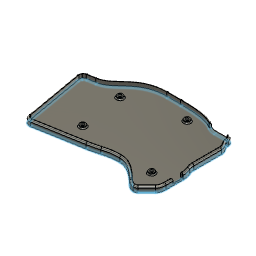
case (Autodesk Fusion 360 design; units mm, degrees)
Autodesk Fusion 360 part; units mm, degrees
note: some values were not read from the file. Set by a fixed rule: the direction of a hole.
sketch "holes" plane through (0, 0, 0) normal (0, 1, 0) x (1, 0, 0)
  circle A0 centre (50.040422, 45.440379) radius 3
  circle A1 centre (43.351531, 91.955525) radius 3
  circle A2 centre (130.099984, 39.118187) radius 3
  circle A3 centre (100.999988, 106.018187) radius 3
  line L0 (119.54041, 105.410769) -> (119.54041, 115.410769)
  line L1 (153.850239, 50.591394) -> (146.676652, 50.591394)
  line L2 (119.54041, 115.410769) -> (139.54041, 115.410769)
  line L3 (146.676652, 50.591394) -> (146.676652, 40.591394)
  line L4 (139.54041, 105.410769) -> (119.54041, 105.410769)
  line L5 (153.850239, 40.591394) -> (153.850239, 50.591394)
  line L6 (146.676652, 40.591394) -> (153.850239, 40.591394)
  line L7 (139.54041, 115.410769) -> (139.54041, 105.410769)
extrude "Extrude7" add sketch "holes" along normal blind 4 contours A0 | A1 | A2 | A3 picked at (49.284643, 47.135619) picked at (42.565449, 90.461331) picked at (132.445357, 39.165571) picked at (101.826227, 105.454867) makes body 1 at (51.274283, 2.666667, -48.174896) makes body 2 at (133.096255, 2.666667, -38.96865) makes body 3 at (46.347802, 2.666667, -91.805987) makes body 4 at (103.996259, 2.666667, -105.86865)
hole "Hole1" at (100.999988, 0, -106.018187) at (43.351531, 0, -91.955525) at (50.040422, 0, -45.440379) at (130.099984, 0, -39.118187) direction (0, 1, 0) diameter 3.3 depth 15 tip angle 180 bodies 1 4 2 3
sketch "outline" plane through (0, 0, 0) normal (0, 1, 0) x (1, 0, 0)
  spline S0 degree 3 poles (147.603738, 59.518008) (146.881991, 61.213684) (146.199862, 62.815653) (146.199862, 66.008223) knots 0 0 0 0 1 1 1 1
  line L0 (146.199862, 66.008223) -> (146.199862, 95.722689)
  spline S1 degree 3 poles (146.199862, 95.722689) (146.199862, 97.999035) (144.934803, 99.77514) (143.818612, 101.342328) (142.857757, 102.691416) (141.949992, 103.965769) (141.949992, 105.358104) knots 2 2 2 2 3 3 3 4 4 4 4
  line L1 (141.949992, 105.358104) -> (141.949992, 107.018123)
  spline S2 degree 3 poles (141.949992, 107.018123) (141.949992, 108.782701) (140.514421, 110.2181) (138.749843, 110.2181) knots 5 5 5 5 6 6 6 6
  line L2 (138.749843, 110.2181) -> (125.549959, 110.2181)
  spline S3 degree 3 poles (125.549959, 110.2181) (121.616005, 110.2181) (119.951335, 111.131223) (117.647255, 112.394711) knots 7 7 7 7 8 8 8 8
  spline S4 degree 3 poles (117.647255, 112.394711) (113.165875, 114.852443) (107.028437, 118.218129) (81.750049, 118.218129) knots 8 8 8 8 9 9 9 9
  line L3 (81.750049, 118.218129) -> (66.990398, 118.217956)
  spline S5 degree 3 poles (66.990398, 118.217956) (48.948261, 117.923228) (40.458988, 110.069833) (32.969219, 103.14084) (27.75056, 98.312914) (23.243542, 94.143457) (16.261884, 93.030863) knots 10 10 10 10 11 11 11 12 12 12 12
  line L4 (16.261884, 93.030863) -> (7.644839, 91.511404)
  ellipse E0 centre (8.763061, 86.940358) end of major axis (11.313219, 82.922603) minor radius 4.306681 (7.644839, 91.511404) -> (5.095124, 89.887041) ccw
  ellipse E1 centre (9.103428, 87.448817) end of major axis (13.733249, 86.415108) minor radius 4.300094 (5.095124, 89.887041) -> (4.440728, 86.935456) ccw
  line L5 (4.440728, 86.935456) -> (15.467273, 24.400083)
  spline S6 degree 3 poles (15.467273, 24.400083) (15.80093, 22.508381) (17.435628, 21.13551) (19.354374, 21.13551) (19.583818, 21.13551) (19.8155, 21.155836) (20.043393, 21.196144) knots 16 16 16 16 17 17 17 18 18 18 18
  line L6 (20.043393, 21.196144) -> (70.514731, 30.095514)
  spline S7 degree 3 poles (70.514731, 30.095514) (75.972968, 31.05773) (79.769808, 32.108828) (83.119819, 33.036248) knots 19 19 19 19 20 20 20 20
  spline S8 degree 3 poles (83.119819, 33.036248) (88.53327, 34.53452) (92.808978, 35.718255) (101.339551, 35.718255) knots 20 20 20 20 21 21 21 21
  spline S9 degree 3 poles (101.339551, 35.718255) (111.773711, 35.629027) (121.148505, 26.837832) (127.99391, 20.41893) knots 21 21 21 21 22 22 22 22
  spline S10 degree 3 poles (127.99391, 20.41893) (128.488281, 19.95522) (128.967149, 19.50598) (129.430515, 19.075687) knots 22 22 22 22 23 23 23 23
  spline S11 degree 3 poles (129.430515, 19.075687) (130.520199, 17.98187) (133.15673, 15.944785) (135.470112, 15.94444) knots 23 23 23 23 24 24 24 24
  spline S12 degree 3 poles (135.470112, 15.94444) (135.470456, 15.94444) (135.470456, 15.94444) (135.470801, 15.94444) (136.374794, 15.94444) (137.172678, 16.252776) (137.793829, 16.851534) knots 24 24 24 24 25 25 25 26 26 26 26
  line L7 (137.793829, 16.851534) -> (147.057001, 26.118152)
  spline S13 degree 3 poles (147.057001, 26.118152) (149.010026, 27.990906) (149.268408, 30.899255) (149.275298, 33.227451) knots 27 27 27 27 28 28 28 28
  line L8 (149.275298, 33.227451) -> (149.275298, 51.551225)
  spline S14 degree 3 poles (149.275298, 51.551225) (149.275298, 55.590944) (148.387153, 57.677293) (147.603738, 59.518008) knots 29 29 29 29 30 30 30 30
  spline S15 degree 3 poles (7.297564, 93.481023) (5.763307, 93.210509) (4.350598, 92.310441) (3.456914, 91.034329) knots 2.78448486 2.78448486 2.78448486 2.78448486 3.50173052 3.50173052 3.50173052 3.50173052
  spline S16 degree 3 poles (3.456914, 91.034329) (2.563151, 89.758126) (2.200589, 88.122569) (2.471108, 86.588186) knots 2.7837328 2.7837328 2.7837328 2.7837328 3.50215444 3.50215444 3.50215444 3.50215444
  line L9 (2.471108, 86.588186) -> (13.497675, 24.052686)
  spline S17 degree 3 poles (13.497675, 24.052686) (13.923121, 21.64058) (15.779485, 19.762796) (18.110966, 19.266153) (18.514055, 19.180288) (18.930917, 19.13551) (19.354374, 19.13551) (19.701936, 19.13551) (20.048463, 19.165998) (20.391728, 19.226712) knots 16 16 16 16 16.85259515 16.85259515 16.85259515 17 17 17 18 18 18 18
  line L10 (20.391728, 19.226712) -> (70.861987, 28.125892)
  spline S18 degree 3 poles (70.861987, 28.125892) (76.409207, 29.103795) (80.303318, 30.1813) (83.6533, 31.108711) knots 19.00000221 19.00000221 19.00000221 19.00000221 19.9999871 19.9999871 19.9999871 19.9999871
  spline S19 degree 3 poles (83.6533, 31.108711) (89.064937, 32.606481) (92.991252, 33.717446) (101.330805, 33.718254) knots 20 20 20 20 20.99965063 20.99965063 20.99965063 20.99965063
  spline S20 degree 3 poles (101.330805, 33.718254) (105.475647, 33.680742) (109.565746, 32.090965) (113.464274, 29.700724) (118.330094, 26.717423) (122.82633, 22.522813) (126.625656, 18.960205) knots 21.00029885 21.00029885 21.00029885 21.00029885 21.44497778 21.44497778 21.44497778 21.99998926 21.99998926 21.99998926 21.99998926
  spline S21 degree 3 poles (126.625656, 18.960205) (127.110442, 18.505485) (127.582537, 18.062588) (128.042517, 17.635267) knots 22 22 22 22 22.98076196 22.98076196 22.98076196 22.98076196
  spline S22 degree 3 poles (128.042517, 17.635267) (128.742667, 16.93793) (129.795646, 16.061685) (131.101379, 15.303235) (132.228147, 14.648739) (133.533208, 14.066903) (135.035069, 13.960088) (135.178323, 13.949899) (135.3233, 13.944462) (135.469814, 13.94444) (135.469864, 13.94444) (135.469913, 13.94444) (135.469963, 13.94444) knots 23.00707695 23.00707695 23.00707695 23.00707695 23.51751165 23.51751165 23.51751165 23.95798579 23.95798579 23.95798579 24 24 24 24.00002146 24.00002146 24.00002146 24.00002146
  spline S23 degree 3 poles (135.469963, 13.94444) (135.470012, 13.94444) (135.470062, 13.94444) (135.470112, 13.94444) (135.470456, 13.94444) (135.470456, 13.94444) (135.470801, 13.94444) (136.751578, 13.94444) (138.036424, 14.394645) (139.007836, 15.25115) (139.06699, 15.303306) (139.125008, 15.356811) (139.181848, 15.411603) (139.186298, 15.415892) (139.190748, 15.420181) (139.195197, 15.42447) knots 23.85591075 23.85591075 23.85591075 23.85591075 24 24 24 25 25 25 25.94260104 25.94260104 25.94260104 26 26 26 26.00716344 26.00716344 26.00716344 26.00716344
  line L11 (139.195197, 15.42447) -> (148.457634, 24.690353)
  spline S24 degree 3 poles (148.457634, 24.690353) (149.759748, 25.946335) (150.461792, 27.512649) (150.832892, 29.003452) (151.208625, 30.512866) (151.271618, 31.980831) (151.27529, 33.221532) (151.275293, 33.222518) (151.275295, 33.223505) (151.275298, 33.224491) knots 27.00207713 27.00207713 27.00207713 27.00207713 27.49794331 27.49794331 27.49794331 28 28 28 28.00042371 28.00042371 28.00042371 28.00042371
  line L12 (151.275298, 33.224491) -> (151.275298, 51.551225)
  spline S25 degree 3 poles (151.275298, 51.551225) (151.275298, 54.695424) (150.746311, 56.906712) (150.130923, 58.59669) (149.898278, 59.235582) (149.658906, 59.796285) (149.444, 60.30123) (149.443996, 60.301239) (149.443992, 60.301249) (149.443988, 60.301258) knots 29 29 29 29 29.7256644 29.7256644 29.7256644 30 30 30 30.00000513 30.00000513 30.00000513 30.00000513
  spline S26 degree 3 poles (149.443988, 60.301258) (149.443984, 60.301268) (149.44398, 60.301277) (149.443976, 60.301287) (148.835826, 61.730075) (148.390307, 62.730144) (148.242825, 64.756889) (148.215259, 65.135702) (148.199862, 65.550338) (148.199862, 66.008223) knots -0.00000557 -0.00000557 -0.00000557 -0.00000557 0 0 0 0.84252605 0.84252605 0.84252605 1 1 1 1
  line L13 (148.199862, 66.008223) -> (148.199862, 95.722689)
  spline S27 degree 3 poles (148.199862, 95.722689) (148.199862, 97.514595) (147.597583, 99.051389) (146.900719, 100.290419) (146.424156, 101.137752) (145.900973, 101.866113) (145.447665, 102.502581) (144.831183, 103.368152) (144.331896, 104.112161) (144.113636, 104.649799) (143.991696, 104.950175) (143.949992, 105.170627) (143.949992, 105.358104) knots 2 2 2 2 2.59387056 2.59387056 2.59387056 3 3 3 3.64156215 3.64156215 3.64156215 4 4 4 4
  line L14 (143.949992, 105.358104) -> (143.949992, 107.018123)
  spline S28 degree 3 poles (143.949992, 107.018123) (143.949992, 109.058672) (142.7586, 110.84858) (141.024034, 111.694202) (140.336548, 112.029359) (139.558567, 112.2181) (138.749843, 112.2181) knots 5 5 5 5 5.71615537 5.71615537 5.71615537 6 6 6 6
  line L15 (138.749843, 112.2181) -> (125.549959, 112.2181)
  spline S29 degree 3 poles (125.549959, 112.2181) (123.526928, 112.2181) (122.32939, 112.46247) (121.264962, 112.851908) (120.422381, 113.16018) (119.627023, 113.590039) (118.60898, 114.148303) knots 7 7 7 7 7.55815924 7.55815924 7.55815924 7.999988 7.999988 7.999988 7.999988
  spline S30 degree 3 poles (118.60898, 114.148303) (116.563943, 115.269867) (113.89365, 116.718364) (109.29887, 117.86132) (103.824782, 119.223006) (95.589531, 120.218129) (81.750049, 120.218129) (81.750045, 120.218129) (81.750041, 120.218129) (81.750037, 120.218129) knots 8 8 8 8 8.4563353 8.4563353 8.4563353 9 9 9 9.00000015 9.00000015 9.00000015 9.00000015
  line L16 (81.750037, 120.218129) -> (66.974052, 120.217956)
  spline S31 degree 3 poles (66.974052, 120.217956) (66.968612, 120.217867) (66.963172, 120.217778) (66.957732, 120.21769) (56.678936, 120.04978) (49.212674, 117.461408) (43.36974, 113.957654) (38.632748, 111.117085) (34.964466, 107.711299) (31.611034, 104.608946) (28.128527, 101.387182) (25.086898, 98.607304) (21.621785, 96.852099) (19.894316, 95.977073) (18.058621, 95.342427) (15.947137, 95.005941) (15.941703, 95.005076) (15.936269, 95.00421) (15.930835, 95.003344) knots 9.99969847 9.99969847 9.99969847 9.99969847 10 10 10 10.55226608 10.55226608 10.55226608 11 11 11 11.66731984 11.66731984 11.66731984 12 12 12 12.00077831 12.00077831 12.00077831 12.00077831
  line L17 (15.930835, 95.003344) -> (7.297564, 93.481023)
  dimension "d20" = 2
extrude "Extrude8" add sketch "outline" along normal blind 6 separate body makes body 5
extrude "Extrude9" cut sketch "outline" along normal blind 2 contours S0 L0 S1 L1 S2 L2 S3 S4 L3 S5 L4 E0 E1 L5 S6 L6 S7 S8 S9 S10 S11 S12 L7 S13 L8 S14 picked at (36.431542, 49.993747) bodies 1 2 3 4
extrude "Extrude10" add sketch "outline" along normal blind 2 contours S0 L0 S1 L1 S2 L2 S3 S4 L3 S5 L4 E0 E1 L5 S6 L6 S7 S8 S9 S10 S11 S12 L7 S13 L8 S14 picked at (36.431542, 49.993747) bodies 1 5 4 2 3
extrude "Extrude11" cut sketch "holes" along normal blind 20 from surface at 2 contours L0 L2 L4 L7 | L1 L3 L5 L6 picked at (126.207077, 108.744102) picked at (149.067847, 47.25806) bodies 1
fillet "Fillet1" radius 1.8 26 edges at (11.6142, 6, -94.242183) (5.137024, 6, -92.634775) (2.527405, 6, -88.908075) (7.984392, 6, -55.320436) (19.354374, 6, -19.13551) (45.626858, 6, -23.676302) (78.081608, 6, -29.636236) (91.394084, 6, -32.974843) (114.903936, 6, -28.777042) (127.343389, 6, -18.287461) (130.994797, 6, -15.365733) (135.470735, 6, -13.94444) (143.826416, 6, -20.057412) (150.840276, 6, -29.033274) (151.275298, 6, -36.907942) (151.275298, 6, -51.071309) (150.666654, 6, -56.856463) (148.561384, 6, -62.69625) (148.199862, 6, -80.865456) (145.447665, 6, -102.502581) (143.949992, 6, -106.188114) (142.683782, 6, -110.414154) (119.088865, 6, -113.886253) (107.924999, 6, -118.181995) (74.362045, 6, -120.218042) (31.607302, 6, -104.605493) on bodies 1 5
chamfer "Chamfer1" distance 1 angle 45 4 edges at (40.554549, 2, -90.870679) (47.24344, 2, -44.355532) (127.303002, 2, -38.033341) (98.203006, 2, -104.933341) on bodies 1
named bodies: "case"
